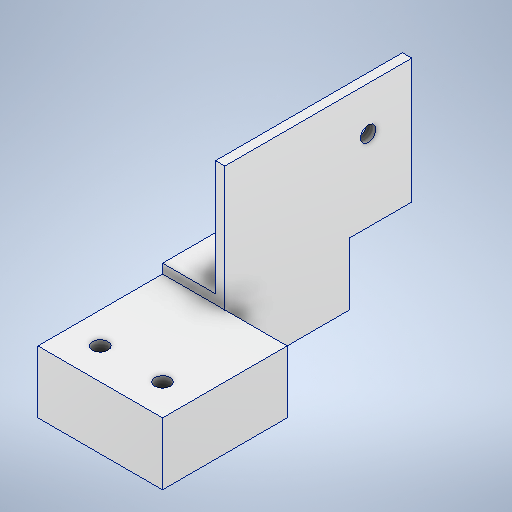
# Autodesk Inventor part: x_bearing_tab
Saved by Autodesk Inventor 2025 (Build 290162000, 162)
## iProperties
Created: 2024-04-25
Part Number: x_bearing_tab
Material: Hliník 6061
Document SubType Name: Modeling
Designer: rader
Density: 2.7 g/cm^3
Appearance: Hliník – plochý
Author: rader
Autodesk Inventor part; units mm, degrees
ref_plane "YZ Plane" through (0, 0, 0) normal (1, 0, 0) x (0, 1, 0)
ref_plane "XZ Plane" through (0, 0, 0) normal (0, 1, 0) x (-1, 0, 0)
ref_plane "XY Plane" through (0, 0, 0) normal (0, 0, 1) x (1, 0, 0)
sketch "Náčrt1" plane through (0, 0, 0) normal (0, 0, 1) x (1, 0, 0)
  line L0 (-14, 0) -> (14, 0) projected
  line L1 (0, 28) -> (0, -28) projected
  line L2 (-10, 20) -> (10, 20)
  line L3 (10, 20) -> (10, -20)
  line L4 (10, -20) -> (-10, -20)
  line L5 (-10, -20) -> (-10, 20)
  point P0 (0, 0)
  dimension "d0" = 20
  dimension "d1" = 40
  constraints: 8 end point, 2 parallel, 1 horizontal, 1 perpendicular, 2 other
  measures "d0" distance of L3.end L4.end
  measures "d1" distance of L2.end L3.end
extrude "Vysunutí1" add sketch "Náčrt1" along normal mid plane 10
sketch "Náčrt2" plane through (0, 0, 5) normal (0, 0, 1) x (1, 0, 0)
  line L0 (-10, -20) -> (10, -20) projected
  line L1 (10, -20) -> (10, 20) projected
  line L2 (10, 20) -> (-10, 20) projected
  line L3 (-10, 20) -> (-10, -20) projected
  line L4 (10, -20) -> (10, 20) projected
  line L5 (0, 20) -> (10, 20)
  line L6 (10, 20) -> (10, 0)
  line L7 (10, 0) -> (0, 0)
  line L8 (0, 0) -> (0, 20)
  point P0 (0, 0)
  constraints: 8 end point, 2 midpoint, 2 parallel, 1 horizontal, 1 perpendicular
extrude "Vysunutí2" cut sketch "Náčrt2" against normal through all contours L7 L8 L2 L1
sketch "Náčrt3" plane through (0, 0, 5) normal (0, 0, 1) x (1, 0, 0)
  line L0 (10, -20) -> (10, 0) projected
  line L1 (-10, -20) -> (10, -20) projected
  point P0 (0, 0)
  point P1 (-5, -15)
  point P2 (5, -15)
  dimension "d6" = 5
  dimension "d7" = 10
  dimension "d8" = 5
  dimension "d9" = 5
  measures "d6" distance from line of L0 point (5, -15)
  measures "d7" distance of point (-5, -15) point (5, -15)
  measures "d8" distance from line of L1 point (-5, -15)
  measures "d9" distance from line of L1 point (5, -15)
hole "Díra1" at (-5, -15, 5) at (5, -15, 5) direction (0, 0, -1) diameter 2.459 depth 5 thread size "M3x0.5" class "6H" standard "ISO Metric profile"
sketch "Náčrt4" plane through (0, 0, 5) normal (0, 0, 1) x (1, 0, 0)
  line L0 (0, 0) -> (-10, 0)
  line L1 (-10, 0) -> (-10, 30)
  line L2 (-10, 30) -> (0, 30)
  line L3 (0, 30) -> (0, 0)
  dimension "d17" = 10
  dimension "d18" = 30
  constraints: 8 end point, 2 parallel, 1 horizontal, 1 perpendicular
  measures "d17" distance of L1.end L2.end
  measures "d18" distance of L0.end L1.end
extrude "Vysunutí3" add sketch "Náčrt4" along normal blind 20
sketch "Náčrt5" plane through (-10, 30, 5) normal (0, 1, 0) x (1, 0, 0)
  line L0 (0, -20) -> (10, -20) projected
  line L1 (0, -20) -> (8.5, -20)
  line L2 (8.5, -20) -> (8.5, -1.5)
  line L3 (8.5, -1.5) -> (0, -1.5)
  line L4 (0, -1.5) -> (0, -20)
  point P0 (10, 5)
  dimension "d21" = 8.5
  dimension "d22" = 18.5
  constraints: 8 end point, 2 parallel, 1 horizontal, 1 perpendicular
  measures "d21" distance of L3.end L2.end
  measures "d22" distance of L2.end L1.end
extrude "Vysunutí4" cut sketch "Náčrt5" against normal through all
sketch "Náčrt6" plane through (0, 0, -5) normal (1, 0, 0) x (0, 0, -1)
  line L0 (0, 20) -> (0, 0) projected
  line L1 (-10, 20) -> (0, 20) projected
  line L2 (-10, 20) -> (-10, 30) projected
  line L3 (-10, 30) -> (-30, 30) projected
  line L4 (-30, 0) -> (-30, 30) projected
  line L5 (-10, 0) -> (-30, 0) projected
  line L6 (-10, 0) -> (0, 0) projected
  point P0 (-5, 0)
  point P1 (-23, 23)
  dimension "d25" = 7
  dimension "d26" = 7
  measures "d25" distance from line of L4 point (-23, 23)
  measures "d26" distance from line of L3 point (-23, 23)
hole "Díra2" at (0, 23, 18) direction (-1, 0, 0) diameter 2.459 end through all thread size "M3x0.5" class "6H" standard "ISO Metric profile"
